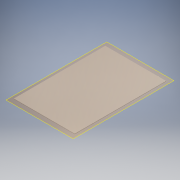
# Autodesk Inventor part: VidrioChico
Saved by Autodesk Inventor 2016 (Build 200138000, 138)
## iProperties
Created: 2018-06-25
Part Number: VidrioChico
Material: Glass
Document SubType Name: Modeling
Designer: damia
Density: 2.18 g/cm^3
Appearance: Clear
Mass: 4179.49 g
Surface Area: 9679.07 cm^2
Volume: 1917.2 cm^3
Author: damia
Autodesk Inventor part; units mm, degrees
ref_plane "YZ Plane" through (0, 0, 0) normal (1, 0, 0) x (0, 1, 0)
ref_plane "XZ Plane" through (0, 0, 0) normal (0, 1, 0) x (-1, 0, 0)
ref_plane "XY Plane" through (0, 0, 0) normal (0, 0, 1) x (1, 0, 0)
ref_plane "Work Plane1" through (-400, 0, 0) normal (0, 0, 1) x (1, 0, 0)
sketch "Sketch1" plane through (-400, 0, 0) normal (0, 0, 1) x (1, 0, 0)
  line L0 (600, 300) -> (-200, 300) projected
  line L1 (-200, 300) -> (-200, -300) projected
  line L2 (-200, -300) -> (600, -300) projected
  line L3 (600, -300) -> (600, 300) projected
  point P0 (400, 0)
extrude "Extrusion1" add sketch "Sketch1" along normal blind 4
chamfer "Chamfer1" distance 1 angle 45 12 edges at (-200, 300, 4) (-600, 0, 4) (200, 0, 4) (-200, -300, 4) (-200, 300, 0) (200, 0, 0) (-600, 0, 0) (-200, -300, 0) (-600, 300, 2) (200, 300, 2) (200, -300, 2) (-600, -300, 2)
body "Solid1"
